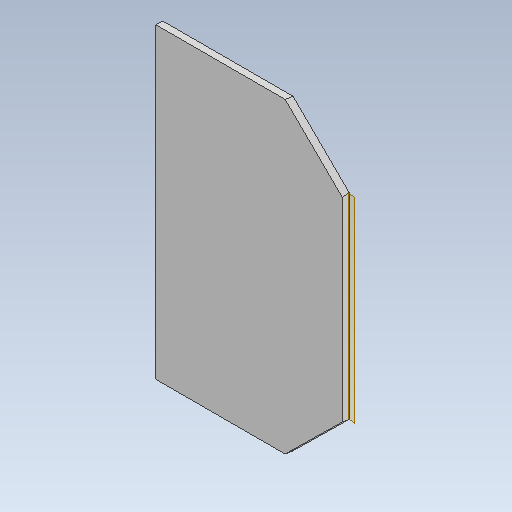
# Autodesk Inventor part: tampa
Saved by Autodesk Inventor 2020 (Build 240168000, 168)
## iProperties
Created: 2020-04-24
Part Number: tampa
Material: Genérico
Document SubType Name: Modeling
Designer: gi-se
Density: 1 g/cm^3
Appearance: Padrão
Author: gi-se
Autodesk Inventor part; units mm, degrees
ref_plane "YZ Plane" through (0, 0, 0) normal (1, 0, 0) x (0, 1, 0)
ref_plane "XZ Plane" through (0, 0, 0) normal (0, 1, 0) x (-1, 0, 0)
ref_plane "XY Plane" through (0, 0, 0) normal (0, 0, 1) x (1, 0, 0)
sketch "Esboço1" plane through (0, 0, 0) normal (0, 1, 0) x (-1, 0, 0)
  line L0 (-83.8742, 0) -> (0, 0)
  line L1 (0, 0) -> (0, 3)
  line L2 (0, 3) -> (-83.8742, 3)
  line L3 (-83.8742, 3) -> (-83.8742, 0)
  dimension "d0" = 3
  constraints: 8 end point, 2 parallel, 1 horizontal, 1 perpendicular
  measures "d0" distance of L1.end L0.end
extrude "Extrusão1" add sketch "Esboço1" along normal blind 138.2
ref_plane "Plano de trabalho1" through (83.8742, 109.1, 0) normal (-0.1736, 0, 0.9848) x (0, -1, 0)
sketch "Esboço2" plane through (83.8742, 109.1, 0) normal (-0.1736, 0, 0.9848) x (0, -1, 0)
  line L0 (0.8787, 5.1213) -> (-31.2213, -26.9787)
  line L1 (79.1213, 5.1213) -> (111.2213, -26.9787)
  line L2 (120.2426, -26.2032) -> (-42, -26.2032)
  line L3 (-42, -26.2032) -> (-42, 2.623)
  line L4 (-42, 2.623) -> (120.2426, 2.623)
  line L5 (120.2426, 2.623) -> (120.2426, -26.2032)
  point P0 (109.1, -82.6)
  point P1 (-30.4458, -26.2032)
  point P2 (-1.6196, 2.623)
  point P3 (81.6196, 2.623)
  point P4 (110.4458, -26.2032)
  constraints: 12 end point
extrude "Extrusão2" cut sketch "Esboço2" along normal blind 13.7 contours L0 L2 L3 L4 | L4 L5 L2 L1
